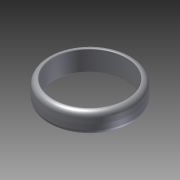
# Autodesk Inventor part: First 09 Wheel_6+375 tread Simple
Saved by Autodesk Inventor 2011 (Build 150239000, 239)
## iProperties
Created: 2010-02-20
Part Number: First 09 Wheel_6+375 tread Simple
Document SubType Name: Modeling
Designer: niemitalo_dan
Density: 1 g/cm^3
Author: niemitalo_dan
Autodesk Inventor part; units mm, degrees
ref_plane "YZ Plane" through (0, 0, 0) normal (1, 0, 0) x (0, 1, 0)
ref_plane "XZ Plane" through (0, 0, 0) normal (0, 1, 0) x (-1, 0, 0)
ref_plane "XY Plane" through (0, 0, 0) normal (0, 0, 1) x (1, 0, 0)
sketch "Sketch1" plane through (0, 0, 0) normal (0, 0, 1) x (1, 0, 0)
  line L0 (-66.6603, -11.4443) -> (-66.6119, -11.4443)
  arc A0 (-68.3474, -19.0449) -> (-66.633, -17.4625) centre (-68.2205, -17.4625) ccw
  arc A1 (-77.1082, -9.779) -> (-68.3474, -19.0449) centre (-67.586, -9.5504) ccw
  line L1 (-77.1082, -9.779) -> (-77.343, 0)
  line L2 (-77.343, 0) -> (-77.1082, 9.779)
  arc A2 (-68.3474, 19.0449) -> (-77.1082, 9.779) centre (-67.586, 9.5504) ccw
  arc A3 (-66.633, 17.4625) -> (-68.3474, 19.0449) centre (-68.2205, 17.4625) ccw
  line L3 (-66.633, 17.4625) -> (-66.633, -17.4625)
  line L4 (0, -29.0182) -> (0, 29.0182) projected
  point P0 (0, 0)
  point P1 (-66.633, 0)
  dimension "d0" = 38.1
  dimension "d1" = 1.5875
  dimension "d2" = 9.525
  dimension "d3" = 19.558
  dimension "d10" = 77.343
  constraints: 8 end point, 8 point on circle, 6 tangent, 4 centre point, 2 equal radius, 2 horizontal alignment, 1 equal length, 1 horizontal, 1 midpoint, 1 vertical
  measures "d1" radius of A3
  measures "d2" radius of A2
  measures "d3" distance of L1.start L2.end
  measures "d10" distance of point (0, 0) L2.start
revolve "Revolution1" add sketch "Sketch1" angle 360 about axis through (0, -10, 0) along (0, 1, 0)
body "Solid1"
